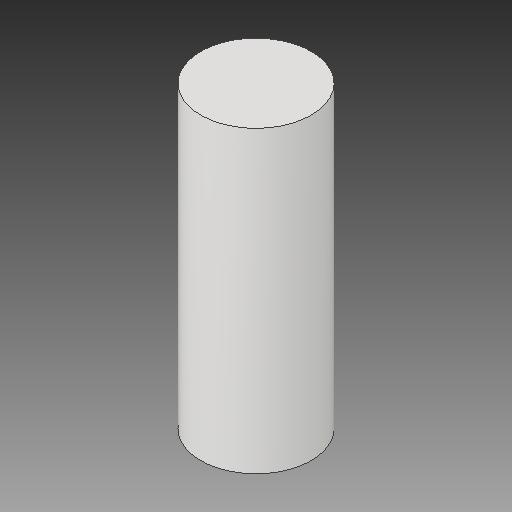
# Autodesk Inventor part: cilindro
Saved by Autodesk Inventor 2018 (Build 220112000, 112)
## iProperties
Created: 2018-04-02
Part Number: cilindro
Material: ABS plástico
Document SubType Name: Modeling
Designer: Ernandes
Density: 1.06 g/cm^3
Appearance: Liso - Branco
Author: Ernandes
Autodesk Inventor part; units mm, degrees
ref_plane "YZ Plane" through (0, 0, 0) normal (1, 0, 0) x (0, 1, 0)
ref_plane "XZ Plane" through (0, 0, 0) normal (0, 1, 0) x (-1, 0, 0)
ref_plane "XY Plane" through (0, 0, 0) normal (0, 0, 1) x (1, 0, 0)
sketch "Esboço1" plane through (0, 0, 0) normal (0, 1, 0) x (-1, 0, 0)
  arc A0 (11.8322, 2) -> (11.8322, -2) centre (0, 0) ccw
  line L0 (-2, 6) -> (-2, 2)
  line L1 (-2, 2) -> (-2, -2)
  line L2 (-2, -2) -> (-2, -6)
  line L3 (2, 2) -> (11.8322, 2)
  line L4 (2, 2) -> (2, 6)
  line L5 (2, 6) -> (-2, 6)
  line L6 (2, -2) -> (2, -6)
  line L7 (2, -6) -> (-2, -6)
  line L8 (11.8322, -2) -> (2, -2)
  constraints: 18 end point, 4 point on line, 2 perpendicular, 2 point on circle, 2 vertical, 1 centre point, 1 coincident
extrude "Extrusão1" add sketch "Esboço1" along normal blind 55
sketch "Esboço2" plane through (0, 55, 0) normal (0, 1, 0) x (1, 0, 0)
  circle A0 centre (0, 0) radius 12
  constraints: 1 centre point, 1 coincident
extrude "Extrusão2" add sketch "Esboço2" along normal blind 10
